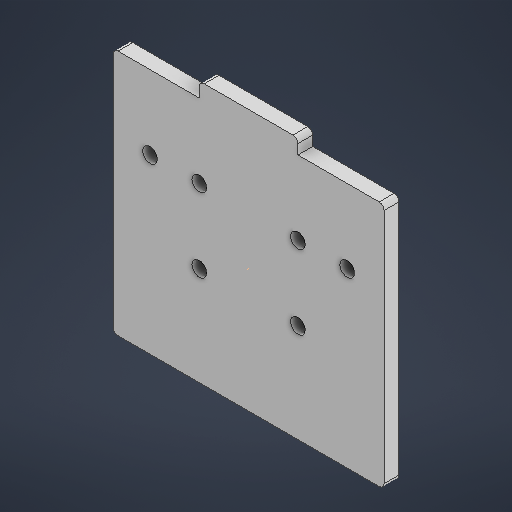
# Autodesk Inventor part: PlacaBaseGarraSTD
Saved by Autodesk Inventor 2026.2 (Build 302298010, 298A)
## iProperties
Created: 2026-04-16
Part Number: PlacaBaseGarraSTD
Material: Genérico
Document SubType Name: Modeling
Designer: Jose Carlos
Density: 1 g/cm^3
Appearance: Valor por defecto
Author: Jose Carlos
Autodesk Inventor part; units mm, degrees
ref_plane "YZ Plane" through (0, 0, 0) normal (1, 0, 0) x (0, 1, 0)
ref_plane "XZ Plane" through (0, 0, 0) normal (0, 1, 0) x (-1, 0, 0)
ref_plane "XY Plane" through (0, 0, 0) normal (0, 0, 1) x (1, 0, 0)
sketch "Boceto1" plane through (0, 0, 0) normal (0, 0, 1) x (1, 0, 0)
  line L0 (-27.5, -25) -> (27.5, -25)
  line L1 (27.5, -25) -> (27.5, 25)
  line L2 (27.5, 25) -> (-27.5, 25)
  line L3 (-27.5, 25) -> (-27.5, -25)
  line L4 (-27.5, -25) -> (27.5, 25) construction
  line L5 (27.5, -25) -> (-27.5, 25) construction
  point P0 (0, 0)
  dimension "d0" = 55
  dimension "d1" = 50
  constraints: 12 end point, 2 midpoint, 2 parallel, 1 horizontal, 1 perpendicular
  measures "d0" distance of L1.end L2.end
  measures "d1" distance of L2.end L0.start
extrude "Extrusión1" add sketch "Boceto1" along normal blind 3
sketch "Boceto2" plane through (0, 0, 3) normal (0, 0, 1) x (1, 0, 0)
  line L0 (-10, 22) -> (10, 22)
  line L1 (10, 22) -> (10, 28)
  line L2 (10, 28) -> (-10, 28)
  line L3 (-10, 28) -> (-10, 22)
  line L4 (27.5, 25) -> (-27.5, 25) construction
  line L5 (-10, 22) -> (10, 28) construction
  line L6 (10, 22) -> (-10, 28) construction
  point P0 (0, 0)
  point P1 (0, 25)
  dimension "d4" = 20
  dimension "d5" = 6
  constraints: 12 end point, 3 midpoint, 2 parallel, 1 horizontal, 1 perpendicular
  measures "d4" distance of L1.end L2.end
  measures "d5" distance of L2.end L0.start
extrude "Extrusión2" add sketch "Boceto2" against normal up to surface (3 mm away)
fillet "Empalme1" radius 1 6 edges at (-27.5, 25, 1.5) (27.5, 25, 1.5) (10, 28, 1.5) (-10, 28, 1.5) (-27.5, -25, 1.5) (27.5, -25, 1.5)
sketch "Boceto3" plane through (0, 0, 0) normal (0, 0, -1) x (-1, 0, 0)
  circle A0 centre (20, 10) radius 1.6 construction
  circle A1 centre (10, 10) radius 1.6 construction
  circle A2 centre (-10, 10) radius 1.6 construction
  circle A3 centre (-20, 10) radius 1.6 construction
  point P0 (0, 0)
  constraints: 4 coincident
hole "Agujero1" at (20, 10, 0) at (10, 10, 0) at (-10, 10, 0) at (-20, 10, 0) direction (0, 0, 1) diameter 3 end through all
sketch "Boceto4" plane through (0, 0, 3) normal (0, 0, 1) x (1, 0, 0)
  line L0 (-26.5, -25) -> (26.5, -25) construction
  line L1 (-27.5, 24) -> (-27.5, -24) construction
  line L2 (0, -35.6) -> (0, 38.6) construction
  line L3 (-10, 25) -> (-26.5, 25) construction
  point P0 (0, 0)
  point P1 (-10, -5)
  dimension "d18" = 10
  dimension "d26" = 30
  measures "d18" distance from line of L2 point (-10, -5)
  measures "d26" distance from line of L3 point (-10, -5)
hole "Agujero2" at (-10, -5, 3) direction (0, 0, -1) diameter 3 end through all
mirror "Simetría1" about plane through (0, 0, 0) normal (1, 0, 0) of "Agujero2"
